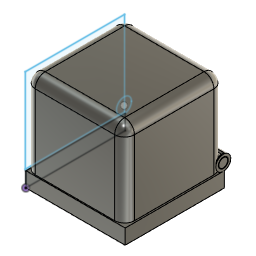
Midterm Asignment v2 (Autodesk Fusion 360 design; units mm, degrees)
Autodesk Fusion 360 part; units mm, degrees
sketch "Sketch1" plane through (0, 0, 0) normal (1, 0, 0) x (0, 1, 0)
  line L0 (0, 0) -> (25.4, 0)
  line L1 (25.4, 0) -> (25.4, 3.81)
  line L2 (25.4, 3.81) -> (0, 3.81)
  line L3 (0, 3.81) -> (0, 0)
  line L4 (25.2468, 4.2339) -> (-0.1532, 4.2339)
  line L5 (-0.1532, 4.2339) -> (-0.1532, 25.8239)
  line L6 (-0.1532, 25.8239) -> (25.2468, 25.8239)
  line L7 (25.2468, 25.8239) -> (25.2468, 4.2339)
  dimension "d1" = 25.4
  dimension "d2" = 3.81
  dimension "d3" = 25.4
  dimension "d4" = 21.59
  constraint horizontal L0
  constraint vertical L1
  constraint horizontal L2
  constraint vertical L3
  constraint coincident L0.start L3.end
  constraint horizontal L4
  constraint vertical L5
  constraint horizontal L6
  constraint vertical L7
  measures "d1" distance of L0.start L0.end
  measures "d2" distance of L0.start L2.end
  measures "d3" distance of L4.start L4.end
  measures "d4" distance of L4.start L6.end
extrude "Extrude1" add sketch "Sketch1" along normal blind 25.4 makes body 1 at (8.4667, 16.7802, 4.2339) makes body 2 at (8.4667, 16.9333, 3.81)
sketch "Sketch2" plane through (0, 0, 0) normal (1, 0, 0) x (0, 1, 0)
  circle A0 centre (25.1015, 5.7134) radius 1.905
  dimension "d7" = 3.81
  measures "d7" diameter of A0
extrude "Extrude2" add sketch "Sketch2" along normal blind 3.81 separate body makes body 3
ref_plane "WorkPlane1" through (25.4, 12.7, 1.905) normal (1, 0, 0) x (0, 0, -1)
sketch "Sketch3" plane through (25.4, 12.7, 1.905) normal (1, 0, 0) x (0, 1, 0)
  circle A0 centre (12.4912, 3.8129) radius 1.905
  dimension "d11" = 3.81
  measures "d11" diameter of A0
shell "Shell1" thickness 1.27 removed faces 1 at (8.4667, 16.7802, 4.2339) on bodies 1
sketch "Sketch4" plane through (0, 0, 0) normal (1, 0, 0) x (0, 1, 0)
ref_plane "WorkPlane2" through (25.4, 12.7, 1.905) normal (1, 0, 0) x (0, 0, -1)
sketch "Sketch5" plane through (25.4, 12.7, 1.905) normal (1, 0, 0) x (0, 1, 0)
  circle A0 centre (12.4081, 3.8023) radius 1.9069
extrude "Extrude4" add sketch "Sketch5" against normal blind 3.81 separate body makes body 4
sketch "Sketch6" plane through (25.4, 0, 0) normal (1, 0, 0) x (0, 1, 0)
  circle A0 centre (25.1081, 5.7073) radius 1.9069
  circle A1 centre (25.1081, 5.7073) radius 1.27
  dimension "d19" = 2.54
  constraint concentric A0 A1
  measures "d19" diameter of A1
extrude "Extrude5" cut sketch "Sketch6" against normal blind 4.064 contours A1 bodies 1 4
sketch "Sketch7" plane through (0, 0, 0) normal (1, 0, 0) x (0, 1, 0)
  circle A0 centre (25.1019, 5.7125) radius 1.27
  dimension "d22" = 2.54
  measures "d22" diameter of A0
extrude "Extrude6" cut sketch "Sketch7" along normal blind 4.064 bodies 1 3
ref_plane "WorkPlane3" through (25.4, 25.1081, 5.7073) normal (1, 0, 0) x (0, 1, 0)
sketch "Sketch8" plane through (0, 0, 0) normal (1, 0, 0) x (0, 1, 0)
  circle A0 centre (25.1036, 5.6991) radius 1.143
  dimension "d26" = 2.286
  measures "d26" diameter of A0
extrude "Extrude7" add sketch "Sketch8" along normal blind 25.4 separate body makes body 5
ref_plane "WorkPlane4" through (23.395, 25.1081, 7.6142) normal (0, 0, 1) x (0, -1, 0)
sketch "Sketch9" plane through (23.395, 25.1081, 7.6142) normal (0, 0, 1) x (1, 0, 0)
  line L0 (-1.5404, 0.4896) -> (1.7777, 0.4896)
  line L1 (1.7777, 0.4896) -> (1.7777, -1.8151)
  line L2 (1.7777, -1.8151) -> (-1.5404, -1.8151)
  line L3 (-1.5404, -1.8151) -> (-1.5404, 0.4896)
  constraint horizontal L0
  constraint vertical L1
  constraint horizontal L2
  constraint vertical L3
extrude "Extrude8" cut sketch "Sketch9" against normal blind 2.286 bodies 4
ref_plane "WorkPlane5" through (2.4292, 25.1015, 7.6184) normal (0, 0, 1) x (0, 1, 0)
sketch "Sketch10" plane through (2.4292, 25.1015, 7.6184) normal (0, 0, 1) x (1, 0, 0)
  line L0 (1.0584, 0.5241) -> (-2.145, 0.5241)
  line L1 (-2.145, 0.5241) -> (-2.145, -1.7685)
  line L2 (-2.145, -1.7685) -> (1.0584, -1.7685)
  line L3 (1.0584, -1.7685) -> (1.0584, 0.5241)
  constraint horizontal L0
  constraint vertical L1
  constraint horizontal L2
  constraint vertical L3
extrude "Extrude9" cut sketch "Sketch10" against normal blind 2.54 bodies 3
combine "Combine1" operation add target body 1 tool bodies 5
copy_body "Body->Comp1" bodies 1 removing the originals makes body 6 in component "Component"
copy_body "Body->Comp2" bodies 4 removing the originals makes body 7 in component "Component'"
combine "Combine2" operation add target body 2 tool bodies 7
fillet "Fillet1" radius 2.54 5 edges at (25.4, -0.1532, 15.0289) (25.4, 25.2468, 16.3968) (25.4, 12.5468, 25.8239) (12.7, 25.2468, 25.8239) (12.7, -0.1532, 25.8239) on bodies 6 in component "Component"
fillet "Fillet2" radius 2.54 6 edges at (1.27, 1.1168, 14.3939) (0, -0.1532, 13.7589) (0, 0.5908, 25.0799) (0, 12.5468, 25.8239) (0, 24.5029, 25.0799) (0, 25.2468, 15.129) on bodies 6 in component "Component"
component "Component" placed x (1, 0, 0) y (0, 1, 0) z (0, 0, 1) at (0, 0.0045, 0.0081)
component "Component'" placed x (1, 0, 0) y (0, 1, 0) z (0, 0, 1) at (0, 0, 0)
